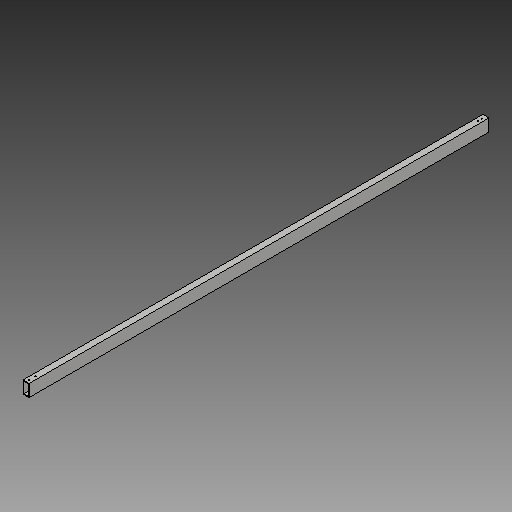
# Autodesk Inventor part: 上昇機構_角柱1
Saved by Autodesk Inventor 2019.4 (Build 234330000, 330)
## iProperties
Created: 2021-12-04
Part Number: 上昇機構_角柱1
Material: アルミニウム 6061
Document SubType Name: Modeling
Designer: 堀川皓史
Density: 2.7 g/cm^3
Appearance: アルミニウム - フラット
Mass: 500.902 g
Surface Area: 1860.08 cm^2
Volume: 185.519 cm^3
Author: 堀川皓史
Autodesk Inventor part; units mm, degrees
ref_plane "YZ Plane" through (0, 0, 0) normal (1, 0, 0) x (0, 1, 0)
ref_plane "XZ Plane" through (0, 0, 0) normal (0, 1, 0) x (-1, 0, 0)
ref_plane "XY Plane" through (0, 0, 0) normal (0, 0, 1) x (1, 0, 0)
sketch "スケッチ1" plane through (0, 0, 0) normal (0, 0, 1) x (1, 0, 0)
  line L0 (7.5, 15) -> (-7.5, 15)
  line L1 (-7.5, 15) -> (-7.5, -15)
  line L2 (-7.5, -15) -> (7.5, -15)
  line L3 (7.5, -15) -> (7.5, 15)
  line L4 (7.5, 15) -> (-7.5, -15) construction
  line L5 (-7.5, 15) -> (7.5, -15) construction
  line L6 (-5.5, 13) -> (5.5, 13)
  line L7 (5.5, 13) -> (5.5, -13)
  line L8 (5.5, -13) -> (-5.5, -13)
  line L9 (-5.5, -13) -> (-5.5, 13)
  point P0 (0, 0)
  dimension "d0" = 15
  dimension "d1" = 30
  dimension "d2" = 2
  constraints: 20 end point, 4 parallel, 2 midpoint, 2 perpendicular, 1 horizontal, 3 other
  measures "d0" distance of L2.end L1.end
  measures "d1" distance of L1.end L0.end
  measures "d2" distance between parallel lines of L0 L6
extrude "押し出し1" add sketch "スケッチ1" along normal blind 1132
sketch "スケッチ2" plane through (-7.5, 15, 1132) normal (0, 1, 0) x (1, 0, 0)
  circle A0 centre (7.5, 1122) radius 1.6
  circle A1 centre (7.5, 1112) radius 1.6
  line L0 (15, 1132) -> (0, 1132) projected
  circle A2 centre (7.5, 7.5) radius 1.6
  circle A3 centre (7.5, 22.5) radius 1.6
  line L1 (15, 0) -> (0, 0) projected
  point P0 (7.5, 1132)
  point P1 (7.5, 1132)
  point P2 (7.5, 0)
  dimension "d5" = 3.2
  dimension "d6" = 3.2
  dimension "d7" = 10
  dimension "d8" = 10
  dimension "d9" = 3.2
  dimension "d10" = 3.2
  dimension "d11" = 15
  dimension "d12" = 7.5
  constraints: 4 centre point, 4 vertical alignment, 2 midpoint
  measures "d5" diameter of A0
  measures "d6" diameter of A1
  measures "d7" distance of A0.centre A1.centre
  measures "d8" distance of point (7.5, 1132) A0.centre
  measures "d9" diameter of A2
  measures "d10" diameter of A3
  measures "d11" distance of A3.centre A2.centre
  measures "d12" distance of point (7.5, 0) A2.centre
extrude "押し出し2" cut sketch "スケッチ2" against normal through all
